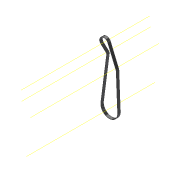
# Autodesk Inventor part: 歯付きベルト
Saved by Autodesk Inventor 2019.4 (Build 234330000, 330)
## iProperties
Created: 2019-11-13
Part Number: 歯付きベルト
Material: Rubber
Document SubType Name: Modeling
Designer: y6tada
Density: 1 g/cm^3
Appearance: Rubber - Black - Version 1.1
CustomPartVersion: 1
Author: y6tada
Autodesk Inventor part; units mm, degrees
ref_plane "YZ Plane" through (0, 0, 0) normal (1, 0, 0) x (0, 1, 0)
ref_plane "XZ Plane" through (0, 0, 0) normal (0, 1, 0) x (-1, 0, 0)
ref_plane "XY Plane" through (0, 0, 0) normal (0, 0, 1) x (1, 0, 0)
sketch "スケッチ パス" plane through (0, 0, 0) normal (0, 0, 1) x (1, 0, 0)
  arc A0 (-17.289552, -70.992395) -> (20.732945, -72.702126) centre (1.649293, -73.457429) ccw
  arc A1 (-4.15897, 29.88981) -> (-5.532073, 33.627969) centre (-8.423003, 30.444806) ccw
  arc A2 (-1.599071, 54.637238) -> (-16.831764, 43.890279) centre (-10.411684, 50.959342) ccw
  arc A3 (17.555663, 7.57581) -> (17.008753, 10.050993) centre (10.399293, 7.292571) ccw
  line L0 (17.555663, 7.57581) -> (20.732945, -72.702126)
  line L1 (-17.289552, -70.992395) -> (-4.15897, 29.88981)
  line L2 (-5.532073, 33.627969) -> (-16.831764, 43.890279)
  line L3 (-1.599071, 54.637238) -> (17.008753, 10.050993)
  constraints: 8 end point, 8 point on circle, 4 centre point
ref_plane "断面平面" through (20.732945, -72.702126, 0) normal (-0.0395476, 0.9992177, 0) x (0, 0, 1)
ref_plane "作業平面2" through (1.649293, -73.457429, 0) normal (-1, 0, 0) x (0, 0, 1)
ref_plane "作業平面3" through (-10.411684, 50.959342, 0) normal (0.6349111, -0.7725852, 0) x (0, 0, 1)
ref_plane "作業平面4" through (10.399293, 7.292571, 0) normal (-0.1994942, 0.979899, 0) x (0, 0, 1)
sketch "断面" plane through (20.732945, -72.702126, 0) normal (-0.0395476, 0.9992177, 0) x (0, 0, 1)
  line L0 (-4, 0.3) -> (4, 0.3)
  line L1 (4, 0.3) -> (4, -0.3)
  line L2 (4, -0.3) -> (-4, -0.3)
  line L3 (-4, -0.3) -> (-4, 0.3)
  line L4 (-4, 0) -> (4, 0) construction
  point P0 (0, 0)
  point P1 (0, 0)
  dimension "d0" = 8
  dimension "d4" = 0.3
  dimension "d5" = 0.3
  constraints: 10 end point, 3 midpoint, 2 parallel, 1 coincident, 1 horizontal, 1 perpendicular, 1 other
  measures "d0" distance between parallel lines of L1 L3
  measures "d4" distance between parallel lines of L2 L4
  measures "d5" distance between parallel lines of L4 L0
sweep "ベルト" add profiles "断面" path "スケッチ パス" path curves L3 A3 L0 A0 L1 A1 L2 A2
equation "\"d4\" = da_a"
equation "\"d5\" = da_a2"
equation "\"da_B\" = 6"
equation "\"da_pb\" = 2.5"
equation "\"da_L\" = 349.7514"
equation "\"da_a\" = 0.3"
equation "\"da_S\" = 1.5"
equation "\"da_Beta\" = 20deg"
equation "\"da_Ht\" = 0.7"
equation "\"da_H\" = 1.3"
equation "\"da_a2\" = 0.3"
body "Solid1"
